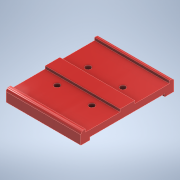
# Autodesk Inventor part: Part1
Saved by Autodesk Inventor 2021 (Build 250183000, 183)
## iProperties
Created: 2022-04-30
Part Number: Part1
Material: Polycarbonate, Clear
Document SubType Name: Modeling
Designer: authe
Density: 1.2 g/cm^3
Appearance: Orange-Red
Author: authe
Autodesk Inventor part; units mm, degrees
ref_plane "YZ Plane" through (0, 0, 0) normal (1, 0, 0) x (0, 1, 0)
ref_plane "XZ Plane" through (0, 0, 0) normal (0, 1, 0) x (-1, 0, 0)
ref_plane "XY Plane" through (0, 0, 0) normal (0, 0, 1) x (1, 0, 0)
sketch "Sketch1" plane through (0, 0, 0) normal (1, 0, 0) x (0, 1, 0)
  line L0 (7, 51) -> (0, 51)
  line L1 (0, 41) -> (0, -41)
  line L2 (0, -51) -> (7, -51)
  line L3 (7, 51) -> (-3, 51)
  line L4 (-3, 51) -> (-3, 41)
  line L5 (-3, 41) -> (0, 41)
  line L6 (7, 41) -> (7, 51)
  line L7 (7, 51) -> (7, 51)
  line L8 (10, 48) -> (10, 46)
  line L9 (10, 46) -> (7, 46)
  line L10 (7, 46) -> (7, 51)
  line L11 (7, 8) -> (10, 8)
  line L12 (10, 8) -> (10, -8)
  line L13 (10, -8) -> (7, -8)
  line L14 (-3, -41) -> (0, -41)
  line L15 (10, -46) -> (7, -46)
  line L16 (7, -51) -> (-3, -51)
  line L17 (-3, -51) -> (-3, -41)
  line L18 (7, -51) -> (0, -51)
  line L19 (7, -41) -> (7, -46)
  line L20 (7, -51) -> (7, -51)
  line L21 (10, -48) -> (10, -46)
  line L22 (7, -46) -> (7, -8)
  line L23 (7, 8) -> (7, 51)
  arc A0 (10, 48) -> (7, 51) centre (7, 48) ccw
  arc A1 (7, -51) -> (10, -48) centre (7, -48) ccw
  point P0 (0, 0)
  point P1 (10, -51)
  point P2 (0, 51)
  dimension "d10" = 10
  dimension "d11" = 10
  dimension "d13" = 5
  dimension "d15" = 43
  dimension "d16" = 59
  dimension "d17" = 102
  dimension "d18" = 13
  dimension "d19" = 3
  dimension "d20" = 3
  constraints: 48 end point, 8 parallel, 4 horizontal, 4 perpendicular, 4 point on circle, 4 tangent, 2 centre point, 2 point on line
  measures "d10" distance of L3.end L4.end
  measures "d11" distance from line of L4 L0.start
  measures "d13" distance of L0.start L9.end
  measures "d15" distance of L0.start L11.start
  measures "d16" distance from line of L3 L13.end
  measures "d17" distance of L7.end L20.end
  measures "d18" distance from line of L17 L21.start
  measures "d19" radius of A1
  measures "d20" radius of A0
extrude "Extrusion1" add sketch "Sketch1" along normal blind 82
sketch "Sketch2" plane through (0, 0, 0) normal (0, 1, 0) x (-1, 0, 0)
  line L0 (0, 51) -> (0, 48) projected
  line L1 (0, 51) -> (0, 17)
  line L2 (0, 41) -> (0, -41) projected
  line L3 (0, 17) -> (-22, 17)
  circle A0 centre (-22, 17) radius 3
  line L4 (0, -41) -> (0, -51) projected
  line L5 (0, -51) -> (0, -17)
  line L6 (0, -17) -> (-22, -17)
  line L7 (0, -41) -> (-82, -41) projected
  line L8 (0, -51) -> (-82, -51) projected
  line L9 (-82, -51) -> (-82, -17)
  line L10 (-82, 41) -> (-82, -41) projected
  line L11 (-82, -17) -> (-60, -17)
  line L12 (-82, 51) -> (-82, 48) projected
  line L13 (-82, 51) -> (-82, 17)
  line L14 (-82, 8) -> (-82, 46) projected
  line L15 (-82, 17) -> (-60, 17)
  circle A1 centre (-22, -17) radius 3
  circle A2 centre (-60, -17) radius 3
  circle A3 centre (-60, 17) radius 3
  point P0 (0, 0)
  dimension "d23" = 34
  dimension "d24" = 22
  dimension "d25" = 6
  dimension "d26" = 34
  dimension "d27" = 22
  dimension "d28" = 34
  dimension "d29" = 22
  dimension "d30" = 34
  dimension "d31" = 22
  dimension "d32" = 6
  dimension "d33" = 6
  dimension "d34" = 6
  constraints: 16 end point, 4 centre point, 4 coincident, 4 point on line, 2 perpendicular, 1 horizontal, 1 parallel
  measures "d23" distance of L0.start L1.end
  measures "d24" distance of L1.end L3.end
  measures "d25" diameter of A0
  measures "d26" distance of L4.end L5.end
  measures "d27" distance of L5.end L6.end
  measures "d28" distance of L8.end L9.end
  measures "d29" distance of L9.end L11.end
  measures "d30" distance of L12.start L13.end
  measures "d31" distance of L13.end L15.end
  measures "d32" diameter of A1
  measures "d33" diameter of A2
  measures "d34" diameter of A3
extrude "Extrusion2" cut sketch "Sketch2" along normal mid plane 62 contours A3 | A2 | A1 | A0
body "Solid1"
